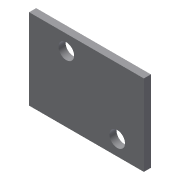
# Autodesk Inventor part: Claw - Arm - Plate 2
Saved by Autodesk Inventor 2015 (Build 190159000, 159)
## iProperties
Created: 2015-02-01
Part Number: Claw - Arm - Plate 2
Material: Generic
Document SubType Name: Sheet Metal
Designer: Tanner
Density: 1 g/cm^3
Sheet Metal Rule: Default
Appearance: Default
Author: Tanner
Autodesk Inventor part; units mm, degrees
ref_plane "YZ Plane" through (0, 0, 0) normal (1, 0, 0) x (0, 1, 0)
ref_plane "XZ Plane" through (0, 0, 0) normal (0, 1, 0) x (-1, 0, 0)
ref_plane "XY Plane" through (0, 0, 0) normal (0, 0, 1) x (1, 0, 0)
sketch "Sketch1" plane through (0, 0, 0) normal (0, 0, 1) x (1, 0, 0)
  line L0 (0, 0) -> (49.53, 0)
  line L1 (49.53, 0) -> (49.53, 34.925)
  line L2 (49.53, 34.925) -> (0, 34.925)
  line L3 (0, 34.925) -> (0, 0)
  dimension "d0" = 49.53
  dimension "d1" = 34.925
  measures "d0" distance of L2.end L1.end
  measures "d1" distance of L1.end L0.end
extrude "Plate1" add sketch "Sketch1" along normal blind 3.048
hole "Hole1" at (38.0365, 6.5532, 3.048) direction (0, 0, -1) diameter 6.731 end through all
hole "Hole2" at (16.0528, 28.3845, 3.048) direction (0, 0, -1) diameter 6.731 end through all
equation "\"d10\" = Thickness"
equation "\"d20\" = Thickness"
equation "\"BendRadius\" = Thickness"
equation "\"BendReliefWidth\" = Thickness"
equation "\"BendReliefDepth\" = 0.5 * Thickness"
equation "\"CornerReliefSize\" = 4 * Thickness"
equation "\"MinimumRemnant\" = 2 * Thickness"
equation "\"TransitionRadius\" = BendRadius"
equation "\"JacobiRadiusSize\" = BendRadius"
equation "\"GapSize\" = Thickness"
equation "\"d2\" = BendRadius"
equation "\"Thickness\" = 3.048"
body "Solid1"
